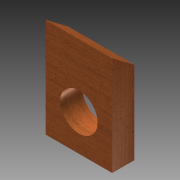
# Autodesk Inventor part: 2p4irsh
Saved by Autodesk Inventor 2014 (Build 180170000, 170)
## iProperties
Company: HERA Project
Created: 2013-12-04
Part Number: 2p4irsh
Material: Wood (Cherry)
Document SubType Name: Modeling
Designer: David DeBoer
Mass: 283.669 g
Surface Area: 501.887 cm^2
Volume: 567.338 cm^3
Density: 0.5 g/cm^3
Description: intermediate rim spar holder
Appearance: Cherry - Natural Low Gloss
Author: David DeBoer
Autodesk Inventor part; units mm, degrees
ref_plane "YZ Plane" through (0, 0, 0) normal (1, 0, 0) x (0, 1, 0)
ref_plane "XZ Plane" through (0, 0, 0) normal (0, 1, 0) x (-1, 0, 0)
ref_plane "XY Plane" through (0, 0, 0) normal (0, 0, 1) x (1, 0, 0)
sketch "Sketch1" plane through (0, 0, 0) normal (1, 0, 0) x (0, 1, 0)
  line L0 (0, 0) -> (170, 0)
  line L1 (0, 0) -> (0, -38)
  line L2 (170, 0) -> (141.3649, -38)
  line L3 (170, 0) -> (170.6921, 0) construction
  line L4 (0, -38) -> (141.3649, -38)
  dimension "d2" = 170
  dimension "d4" = 38
  dimension "d26" = 127
  constraints: 10 end point, 2 horizontal, 1 parallel, 1 perpendicular
  measures "d2" distance of L0.start L0.end
  measures "d4" distance of L0.start L1.end
  measures "d26" angle of L2 L3
extrude "Extrusion1" add sketch "Sketch1" along normal blind 114
sketch "Sketch4" plane through (0, 170, 0) normal (0, 0.7986355, -0.601815) x (1, 0, 0)
  line L0 (0, 47.5812) -> (114, 47.5812) projected
  circle A0 centre (76, 23.7906) radius 2.921
  line L1 (0, 0) -> (0, 47.5812) projected
  line L2 (0, 0) -> (114, 0) projected
  line L3 (76, 23.7906) -> (38, 23.7906) construction
  line L4 (57, 47.5812) -> (57, 0) construction
  point P0 (0, 102.3086)
  point P1 (57, 23.7906)
  dimension "d30" = 38
  dimension "d42" = 38
  constraints: 4 end point, 4 midpoint, 1 centre point, 1 horizontal, 1 parallel, 1 other
  measures "d30" distance of L3.start L3.end
  measures "d42" distance from line of L1 L3.end
hole "Hole2" at (38, 155.6825, -19) at (76, 155.6825, -19) direction (0, -0.7986355, 0.601815) diameter 1 depth 25.4 tip angle 118
sketch "Sketch5" plane through (0, 0, 0) normal (0, 0, 1) x (1, 0, 0)
  line L0 (0, 170) -> (114, 170) projected
  circle A0 centre (57, 62) radius 32
  dimension "d44" = 64
  dimension "d45" = 108
  constraints: 1 centre point
  measures "d44" diameter of A0
  measures "d45" distance from line of A0.centre L0
hole "Hole3" at (57, 62, 0) direction (0, 0, -1) diameter 64 end through all
body "Solid1"
